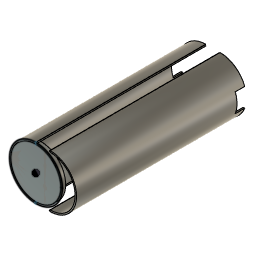
2022_09_15_MoldCylinder v1 (Autodesk Fusion 360 design; units mm, degrees)
Autodesk Fusion 360 part; units mm, degrees
other "Base Mesh Feature1"
sketch "Sketch1" plane through (0, 0, 0) normal (0, 1, 0) x (1, 0, 0)
  circle A0 centre (0, 0) radius 26.5
  circle A1 centre (0, 0) radius 28
  line L0 (0.0082, -28) -> (0.0082, -26.5)
  line L1 (0.0082, 26.5) -> (0.0082, 28)
  line L2 (0.0082, 27.25) -> (-1, 27.25)
  line L3 (-1, 27.25) -> (0.0082, 26.5)
  line L4 (-1, 27.25) -> (0.0082, 28)
  line L5 (0.0082, -27.25) -> (-1, -27.25)
  line L6 (-1, -27.25) -> (0.0082, -28)
  line L7 (-1, -27.25) -> (0.0082, -26.5)
  dimension "d1" = 53
  dimension "d2" = 56
  constraint coincident A0.centre A1.centre
  constraint coincident A1 L0.start
  constraint coincident A0 L0.end
  constraint vertical L0
  constraint coincident A0 L1.start
  constraint coincident A1 L1.end
  constraint parallel L0 L1
  constraint midpoint L1 L2.start
  constraint perpendicular L1 L2
  constraint midpoint L0 L5.start
  constraint perpendicular L0 L5
  measures "d1" diameter of A0
  measures "d2" diameter of A1
extrude "Extrude1" add sketch "Sketch1" along normal blind 180 contours A0 A1 L0 L1 | L1 L2 L3 | L0 L5 L7 | L1 L2 L4 | L0 L5 L6 makes body 1
extrude "Extrude2" add sketch "Sketch1" along normal blind 180 separate body contours A0 A1 L3 L4 L6 L7 makes body 2
extrude "Extrude3" add sketch "Sketch1" along normal blind 5 contours A0 bodies 2
move_body "Move1" bodies 1 to x (1, 0, 0) y (0, 1, 0) z (0, 0, 1) at (15, 0, 0)
sketch "Sketch2" plane through (0, 0, 0) normal (1, 0, 0) x (0, 1, 0)
  line L0 (190, -10) -> (170, -10)
  line L1 (170, -10) -> (170, 10)
  line L2 (170, 10) -> (190, 10)
  line L3 (190, 10) -> (190, -10)
  constraint horizontal L0
  constraint vertical L1
  constraint horizontal L2
  constraint vertical L3
extrude "Extrude4" cut sketch "Sketch2" along normal blind 70 and the other way blind 50 bodies 1 2
